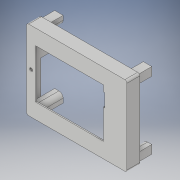
# Autodesk Inventor part: case_top
Saved by Autodesk Inventor 2019 (Build 230136000, 136)
## iProperties
Created: 2019-03-26
Part Number: case_top
Material: Generic
Document SubType Name: Modeling
Designer: janza
Density: 1 g/cm^3
Appearance: Default
Author: janza
## iProperties of the stored document case_top_3DPrint.ipt
Created: 2019-03-30
Part Number: case_top_3DPrint
Material: Generic
Document SubType Name: Modeling
Designer: janza
Density: 1 g/cm^3
Appearance: Default
Author: janza
Autodesk Inventor part; units mm, degrees
ref_plane "YZ Plane" through (0, 0, 0) normal (1, 0, 0) x (0, 1, 0)
ref_plane "XZ Plane" through (0, 0, 0) normal (0, 1, 0) x (-1, 0, 0)
ref_plane "XY Plane" through (0, 0, 0) normal (0, 0, 1) x (1, 0, 0)
sketch "vrsek" plane through (0, 0, 0) normal (0, 0, 1) x (1, 0, 0)
  line L0 (0, 0) -> (92, 0)
  line L1 (92, 0) -> (92, 72)
  line L2 (92, 72) -> (0, 72)
  line L3 (0, 72) -> (0, 0)
  dimension "d0" = 92
  dimension "d1" = 72
  constraints: 8 end point, 2 parallel, 1 horizontal, 1 perpendicular
  measures "d0" distance of L2.end L1.end
  measures "d1" distance of L1.end L0.end
extrude "Extrusion1" add sketch "vrsek" along normal blind 1.2 and the other way blind 0.4
sketch "displej_vyrez" plane through (0, 0, 1.2) normal (0, 0, 1) x (1, 0, 0)
  line L0 (0, 72) -> (0, 0) projected
  line L1 (92, 0) -> (92, 72) projected
  line L2 (0, 36) -> (7, 36)
  line L3 (7, 36) -> (7, 59.15)
  line L4 (7, 59.15) -> (71.2, 59.15)
  line L5 (71.2, 59.15) -> (71.2, 53.35)
  line L6 (71.2, 53.35) -> (72.7, 53.35)
  line L7 (72.7, 53.35) -> (72.7, 40.95)
  line L8 (72.7, 40.95) -> (71.2, 40.95)
  line L9 (7, 36) -> (7, 12.85)
  line L10 (7, 12.85) -> (71.2, 12.85)
  line L11 (71.2, 12.85) -> (71.2, 40.95)
  line L12 (0, 0) -> (92, 0) projected
  dimension "d4" = 7
  dimension "d5" = 23.15
  dimension "d6" = 64.2
  dimension "d7" = 5.8
  dimension "d8" = 1.5
  dimension "d9" = 12.4
  dimension "d10" = 1.5
  dimension "d11" = 23.15
  dimension "d12" = 36
  constraints: 20 end point, 6 perpendicular, 1 horizontal, 1 midpoint, 1 parallel, 1 point on line, 1 vertical
  measures "d4" distance of L2.start L2.end
  measures "d5" distance of L2.end L3.end
  measures "d6" distance of L3.end L4.end
  measures "d7" distance of L4.end L5.end
  measures "d8" distance of L5.end L6.end
  measures "d9" distance of L6.end L7.end
  measures "d10" distance of L7.end L8.end
  measures "d11" distance of L2.end L9.end
  measures "d12" distance between parallel lines of L12 L2
extrude "Extrusion2" cut sketch "displej_vyrez" against normal blind 3
sketch "resetTL_zarez_vedeni" plane through (0, 0, 1.2) normal (0, 0, 1) x (1, 0, 0)
  line L0 (0.5, 40.85) -> (5, 40.85)
  line L1 (5, 40.85) -> (5, 33.85)
  line L2 (5, 33.85) -> (0.5, 33.85)
  line L3 (0.5, 33.85) -> (0.5, 40.85)
  line L4 (0, 0) -> (92, 0) projected
  line L5 (7, 12.85) -> (7, 59.15) projected
  line L6 (71.2, 12.85) -> (7, 12.85) projected
  dimension "d15" = 4.5
  dimension "d16" = 7
  dimension "d19" = 2
  dimension "d20" = 21
  constraints: 8 end point, 2 parallel, 1 horizontal, 1 perpendicular
  measures "d15" distance of L1.end L2.end
  measures "d16" distance of L0.end L1.end
  measures "d19" distance between parallel lines of L5 L1
  measures "d20" distance between parallel lines of L6 L2
sketch "resetTL_vnitrek_vybrani" plane through (0, 0, -0.4) normal (0, 0, -1) x (-1, 0, 0)
  line L0 (-5, 33.85) -> (-0.5, 33.85) projected
  line L1 (-5, 40.85) -> (-5, 33.85) projected
  line L2 (-0.5, 40.85) -> (-5, 40.85) projected
  line L3 (-0.5, 33.85) -> (-0.5, 40.85) projected
  point P0 (0, 0)
extrude "Extrusion3" cut sketch "resetTL_vnitrek_vybrani" against normal blind 0.9
sketch "resetTL_dira" plane through (0, 0, 0.5) normal (0, 0, -1) x (-1, 0, 0)
  line L0 (-5, 33.85) -> (-5, 40.85) projected
  circle A0 centre (-2.7431, 37.35) radius 1.5
  point P0 (0, 0)
  dimension "d23" = 3
  constraints: 1 centre point
  measures "d23" diameter of A0
extrude "Extrusion4" cut sketch "resetTL_dira" against normal blind 2
sketch "spojeni_srouby" plane through (0, 0, -0.4) normal (0, 0, -1) x (-1, 0, 0)
  line L0 (-92, 72) -> (0, 72)
  line L1 (-8, 68) -> (-8, 72)
  line L2 (-4, 72) -> (0, 72)
  line L3 (-8, 72) -> (0, 72)
  line L4 (0, 72) -> (0, 71.7851)
  line L5 (0, 0) -> (-92, 0)
  line L6 (0, 72) -> (0, 0)
  line L7 (0, 0) -> (0, 36)
  line L8 (0, 36) -> (-92, 36)
  line L9 (-92, 0) -> (-92, 72)
  line L10 (-46, 36) -> (-46, 18.5898)
  line L11 (-92, 0) -> (0, 0)
  line L12 (-8, 4) -> (-8, 0)
  line L13 (-4, 0) -> (0, 0)
  line L14 (-8, 0) -> (0, 0)
  line L15 (0, 0) -> (0, 0.2149)
  line L16 (0, 0) -> (0, 72)
  line L17 (-84, 68) -> (-84, 72)
  line L18 (-88, 72) -> (-92, 72)
  line L19 (-84, 72) -> (-92, 72)
  line L20 (-92, 72) -> (-92, 71.7851)
  line L21 (-84, 4) -> (-84, 0)
  line L22 (-88, 0) -> (-92, 0)
  line L23 (-84, 0) -> (-92, 0)
  line L24 (-92, 0) -> (-92, 0.2149)
  line L25 (-92, 72) -> (-92, 72)
  line L26 (-92, 0) -> (-92, 0)
  line L27 (-92, 0) -> (-84, 0)
  line L28 (-88, 64) -> (-92, 64)
  line L29 (-92, 64) -> (-92, 72)
  arc A0 (-88, 64) -> (-84, 68) centre (-88, 68) ccw
  line L30 (-88, 8) -> (-92, 8)
  arc A1 (-84, 4) -> (-88, 8) centre (-88, 4) ccw
  line L31 (-4, 8) -> (0, 8)
  arc A2 (-4, 8) -> (-8, 4) centre (-4, 4) ccw
  line L32 (-4, 64) -> (0, 64)
  arc A3 (-8, 68) -> (-4, 64) centre (-4, 68) ccw
  line L33 (0, 72) -> (0, 56.55)
  line L34 (0, 72) -> (0, 64)
  line L35 (0, 8) -> (0, 0)
  line L36 (-92, 0) -> (-92, 8)
  line L37 (-92, 64) -> (-92, 72)
  line L38 (-84, 72) -> (-92, 72)
  line L39 (0, 72) -> (-8, 72)
  constraints: 80 end point, 24 symmetric about line, 8 perpendicular, 8 point on circle, 7 collinear, 6 point on line, 4 centre point, 4 tangent, 3 midpoint, 3 vertical
extrude "Extrusion7" add sketch "spojeni_srouby" along normal blind 23.5 contours L0 L17 A0 L28 L9 | L0 L4 L6 L32 A3 L1 | L30 A1 L21 L5 L9 | L6 L5 L12 A2 L31
sketch "diry_zavitova_vlozka" plane through (0, 0, -23.9) normal (0, 0, -1) x (-1, 0, 0)
  arc A0 (-84, 4) -> (-88, 8) centre (-88, 4) ccw projected
  arc A1 (-4, 8) -> (-8, 4) centre (-4, 4) ccw projected
  arc A2 (-8, 68) -> (-4, 64) centre (-4, 68) ccw projected
  arc A3 (-88, 64) -> (-84, 68) centre (-88, 68) ccw projected
  point P0 (0, 0)
  constraints: 4 coincident
hole "Hole1" at (88, 4, -23.9) at (4, 4, -23.9) at (4, 68, -23.9) at (88, 68, -23.9) direction (0, 0, 1) diameter 3.5 depth 12 countersink diameter 3.85 countersink angle 10
sketch "Sketch10" plane through (0, 0, -0.4) normal (0, 0, -1) x (-1, 0, 0)
  line L0 (-71.2, 59.15) -> (-7, 59.15) projected
  line L1 (-7, 59.15) -> (-7, 12.85) projected
  line L2 (-7, 12.85) -> (-71.2, 12.85) projected
  line L3 (-71.2, 12.85) -> (-71.2, 40.95) projected
  line L4 (-71.2, 40.95) -> (-72.7, 40.95) projected
  line L5 (-72.7, 40.95) -> (-72.7, 53.35) projected
  line L6 (-72.7, 53.35) -> (-71.2, 53.35) projected
  line L7 (-84, 4) -> (-84, 0) projected
  line L8 (-84, 0) -> (-8, 0) projected
  line L9 (-8, 0) -> (-8, 4) projected
  arc A0 (-4, 8) -> (-8, 4) centre (-4, 4) ccw projected
  line L10 (-4, 8) -> (0, 8) projected
  line L11 (0, 8) -> (0, 64) projected
  line L12 (0, 64) -> (-4, 64) projected
  arc A1 (-8, 68) -> (-4, 64) centre (-4, 68) ccw projected
  line L13 (-8, 68) -> (-8, 72) projected
  line L14 (-8, 72) -> (-84, 72) projected
  line L15 (-84, 72) -> (-84, 68) projected
  arc A2 (-88, 64) -> (-84, 68) centre (-88, 68) ccw projected
  line L16 (-88, 64) -> (-92, 64) projected
  line L17 (-92, 64) -> (-92, 8) projected
  line L18 (-92, 8) -> (-88, 8) projected
  arc A3 (-84, 4) -> (-88, 8) centre (-88, 4) ccw projected
  line L19 (-0.5, 40.85) -> (-0.5, 33.85) projected
  line L20 (-0.5, 33.85) -> (-5, 33.85) projected
  line L21 (-5, 33.85) -> (-5, 40.85) projected
  line L22 (-5, 40.85) -> (-0.5, 40.85) projected
  line L23 (-7, 12.85) -> (-71.2, 12.85) projected
  line L24 (-71.2, 12.85) -> (-71.2, 40.95) projected
  line L25 (-71.2, 40.95) -> (-72.7, 40.95) projected
  line L26 (-72.7, 40.95) -> (-72.7, 53.35) projected
  line L27 (-72.7, 53.35) -> (-71.2, 53.35) projected
  line L28 (-71.2, 53.35) -> (-71.2, 59.15) projected
  line L29 (-71.2, 59.15) -> (-7, 59.15) projected
  line L30 (-7, 59.15) -> (-7, 12.85) projected
  line L31 (-73.7, 61.65) -> (-73.7, 55.85)
  line L32 (-73.7, 55.85) -> (-75.2, 55.85)
  line L33 (-75.2, 55.85) -> (-75.2, 38.45)
  line L34 (-75.2, 38.45) -> (-73.7, 38.45)
  line L35 (-73.7, 38.45) -> (-73.7, 10.35)
  line L36 (-73.7, 10.35) -> (-4.5, 10.35)
  line L37 (-4.5, 10.35) -> (-4.5, 61.65)
  line L38 (-4.5, 61.65) -> (-73.7, 61.65)
  point P0 (0, 0)
  dimension "d58" = 2.5
  constraints: 16 end point, 7 other
  measures "d58" distance between parallel lines of L28 L31
extrude "Extrusion8" cut sketch "Sketch10" against normal blind 0.5 contours L37 L20 L21 L22 | L22 L21 L20 L37 L36 L35 L34 L33 L32 L31 L38
sketch "dira_RJ45" plane through (0, 0, -0.4) normal (0, 0, -1) x (-1, 0, 0)
  line L0 (1.6, 39.75) -> (0, 39.75)
  line L1 (0, 39.75) -> (0, 56.55)
  line L2 (0, 56.55) -> (1.6, 56.55)
  line L3 (1.6, 56.55) -> (1.6, 39.75)
  line L4 (-84, 0) -> (-8, 0) projected
  line L5 (0, 8) -> (0, 64) projected
  line L6 (0, 72) -> (-8, 72) projected
  point P0 (0, 0)
  dimension "d61" = 1.6
  dimension "d62" = 16.8
  dimension "d64" = 0
  dimension "d74" = 15.45
  constraints: 8 end point, 2 parallel, 1 horizontal, 1 perpendicular
  measures "d61" distance of L1.end L2.end
  measures "d62" distance of L0.end L1.end
  measures "d64" distance between parallel lines of L5 L1
  measures "d74" distance between parallel lines of L6 L2
extrude "Extrusion9" add sketch "dira_RJ45" along normal blind 17.6 and the other way blind 1.6
sketch "Sketch12" plane through (0, 0, -0.4) normal (0, 0, -1) x (-1, 0, 0)
  line L0 (0, 56.55) -> (0, 64) projected
  line L1 (0, 64) -> (0, 72) projected
  line L2 (0, 72) -> (-8, 72) projected
  line L3 (-8, 72) -> (-84, 72) projected
  line L4 (-84, 72) -> (-92, 72) projected
  line L5 (-92, 72) -> (-92, 64) projected
  line L6 (-92, 64) -> (-92, 8) projected
  line L7 (-92, 8) -> (-92, 0) projected
  line L8 (-92, 0) -> (-84, 0) projected
  line L9 (-84, 0) -> (-8, 0) projected
  line L10 (-8, 0) -> (0, 0) projected
  line L11 (0, 0) -> (0, 8) projected
  line L12 (0, 8) -> (0, 39.75) projected
  line L13 (1.6, 56.55) -> (1.6, 63)
  line L14 (1.6, 63) -> (1.6, 73.6)
  line L15 (1.6, 73.6) -> (-8, 73.6)
  line L16 (-8, 73.6) -> (-84, 73.6)
  line L17 (-84, 73.6) -> (-93.6, 73.6)
  line L18 (-93.6, 73.6) -> (-93.6, 64)
  line L19 (-93.6, 64) -> (-93.6, 8)
  line L20 (-93.6, 8) -> (-93.6, -1.6)
  line L21 (-93.6, -1.6) -> (-84, -1.6)
  line L22 (-84, -1.6) -> (-8, -1.6)
  line L23 (-8, -1.6) -> (1.6, -1.6)
  line L24 (1.6, -1.6) -> (1.6, 7)
  line L25 (1.6, 7) -> (1.6, 39.75)
  line L26 (1.6, 56.55) -> (0, 56.55) projected
  line L27 (0, 56.55) -> (1.6, 56.55)
  line L28 (0, 39.75) -> (0, 56.55) projected
  line L29 (1.6, 39.75) -> (0, 39.75)
  constraints: 30 end point, 1 collinear, 1 horizontal, 12 other
extrude "Extrusion10" add sketch "Sketch12" along normal blind 10.5 and the other way blind 1.6 contours L0 L1 L2 L3 L4 L5 L6 L7 L8 L9 L10 L11 L12 L29 L25 L24 L23 L22 L21 L20 L19 L18 L17 L16 L15 L14 L13 L26
fillet "Fillet1" radius 2 4 edges at (-1.6, 73.6, -4.85) (93.6, 73.6, -4.85) (93.6, -1.6, -4.85) (-1.6, -1.6, -4.85)
body "Solid1"
